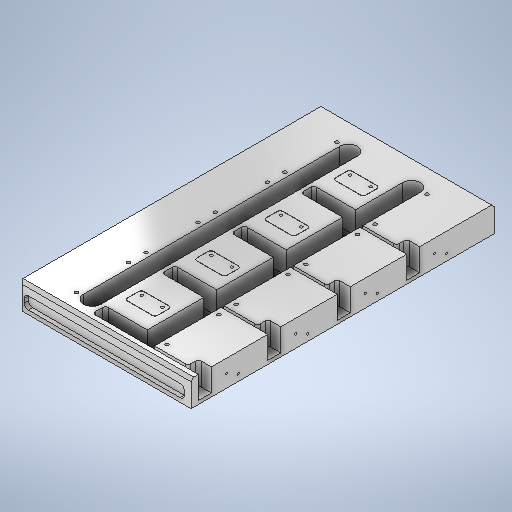
# Autodesk Inventor part: Assembly Plate
Saved by Autodesk Inventor 2025 (Build 290162000, 162)
## iProperties
Created: 2022-03-23
Part Number: Assembly Plate
Material: Generic
Document SubType Name: Modeling
Designer: Caleb
Density: 1 g/cm^3
Appearance: Aluminum - Dark
Author: Caleb
Autodesk Inventor part; units mm, degrees
ref_plane "YZ Plane" through (0, 0, 0) normal (1, 0, 0) x (0, 1, 0)
ref_plane "XZ Plane" through (0, 0, 0) normal (0, 1, 0) x (-1, 0, 0)
ref_plane "XY Plane" through (0, 0, 0) normal (0, 0, 1) x (1, 0, 0)
sketch "Sketch1" plane through (0, 0, 0) normal (0, 1, 0) x (-1, 0, 0)
  line L0 (-63.5, -111) -> (63.5, -111)
  line L1 (63.5, -111) -> (63.5, 111)
  line L2 (63.5, 111) -> (-63.5, 111)
  line L3 (-63.5, 111) -> (-63.5, -111)
  line L4 (-63.5, -111) -> (63.5, 111) construction
  line L5 (63.5, -111) -> (-63.5, 111) construction
  point P0 (0, 0)
  dimension "d0" = 127
  dimension "d1" = 222
  constraints: 12 end point, 2 midpoint, 2 parallel, 1 horizontal, 1 perpendicular
  measures "d0" distance of L2.end L1.end
  measures "d1" distance of L1.end L0.end
extrude "Extrusion1" add sketch "Sketch1" along normal blind 19.05
sketch "Sketch8" plane through (63.5, 0, -111) normal (0, 0, -1) x (-1, 0, 0)
  line L0 (119, 3) -> (8, 3)
  line L1 (5, 6) -> (5, 9)
  line L2 (8, 12) -> (119, 12)
  line L3 (122, 9) -> (122, 6)
  line L4 (122, 3) -> (5, 12) construction
  line L5 (5, 3) -> (122, 12) construction
  line L6 (0, 0) -> (0, 19.05) projected
  line L7 (127, 0) -> (127, 19.05) projected
  line L8 (0, 0) -> (127, 0) projected
  arc A0 (8, 12) -> (5, 9) centre (8, 9) ccw
  arc A1 (5, 6) -> (8, 3) centre (8, 6) ccw
  arc A2 (119, 3) -> (122, 6) centre (119, 6) ccw
  arc A3 (122, 9) -> (119, 12) centre (119, 9) ccw
  point P0 (63.5, 0)
  point P1 (63.5, 7.5)
  point P2 (0, 15.875)
  point P3 (127, 15.875)
  dimension "d77" = 9
  dimension "d78" = 5
  dimension "d79" = 5
  dimension "d80" = 3
  dimension "d83" = 3
  constraints: 12 end point, 8 point on circle, 8 point on line, 8 tangent, 4 centre point, 3 equal radius, 2 midpoint, 2 parallel, 1 horizontal, 1 perpendicular
  measures "d77" distance of L5.start L4.end
  measures "d78" distance between parallel lines of L6 L1
  measures "d79" distance between parallel lines of L7 L3
  measures "d80" distance between parallel lines of L8 L0
  measures "d83" radius of A0
extrude "Extrusion4" cut sketch "Sketch8" against normal blind 3
sketch "Sketch9" plane through (63.5, 0, 111) normal (0, 0, 1) x (1, 0, 0)
  line L0 (-8, 3) -> (-119, 3)
  line L1 (-122, 6) -> (-122, 9)
  line L2 (-119, 12) -> (-8, 12)
  line L3 (-5, 9) -> (-5, 6)
  line L4 (-5, 3) -> (-122, 12) construction
  line L5 (-122, 3) -> (-5, 12) construction
  arc A0 (-119, 12) -> (-122, 9) centre (-119, 9) ccw
  arc A1 (-122, 6) -> (-119, 3) centre (-119, 6) ccw
  arc A2 (-8, 3) -> (-5, 6) centre (-8, 6) ccw
  arc A3 (-5, 9) -> (-8, 12) centre (-8, 9) ccw
  line L6 (-127, 0) -> (0, 0) projected
  line L7 (-127, 0) -> (-127, 19.05) projected
  line L8 (0, 0) -> (0, 19.05) projected
  point P0 (63.5, 0)
  point P1 (-63.5, 7.5)
  dimension "d84" = 9
  dimension "d88" = 3
  dimension "d89" = 3
  dimension "d93" = 5
  dimension "d94" = 5
  constraints: 12 end point, 8 point on circle, 8 point on line, 8 tangent, 4 centre point, 3 equal radius, 2 midpoint, 2 parallel, 1 horizontal, 1 perpendicular
  measures "d84" distance of L5.start L4.end
  measures "d88" radius of A0
  measures "d89" distance between parallel lines of L6 L0
  measures "d93" distance between parallel lines of L7 L1
  measures "d94" distance between parallel lines of L8 L3
extrude "Extrusion5" cut sketch "Sketch9" against normal blind 3
sketch "Sketch10" plane through (0, 19.05, 0) normal (0, 1, 0) x (1, 0, 0)
  line L0 (63.5, -111) -> (63.5, 111) projected
  line L1 (-63.5, -111) -> (63.5, -111) projected
  line L2 (-63.5, 111) -> (-63.5, -111) projected
  line L3 (13.3831, -79.25) -> (-9.5437, -79.25) construction
  line L4 (0, -90.2687) -> (0, -62.9539) construction
  line L5 (13.3831, -28.45) -> (-9.5437, -28.45) construction
  line L6 (0, -39.4687) -> (0, -12.1539) construction
  line L7 (13.3831, 22.35) -> (-9.5437, 22.35) construction
  line L8 (0, 11.3313) -> (0, 38.6461) construction
  line L9 (13.3831, 73.15) -> (-9.5437, 73.15) construction
  line L10 (0, 62.1313) -> (0, 89.4461) construction
  point P0 (23, -96.75)
  point P1 (23, -85.0833)
  point P2 (-23, -96.75)
  point P3 (-23, -85.0833)
  point P4 (23, -73.4167)
  point P5 (-23, -73.4167)
  point P6 (23, -61.75)
  point P7 (-23, -61.75)
  point P8 (0, -79.25)
  point P9 (33, -98.25)
  point P10 (33, -60.25)
  point P11 (-33, -98.25)
  point P12 (-33, -60.25)
  point P13 (0, -28.45)
  point P14 (-33, -9.45)
  point P15 (-33, -47.45)
  point P16 (33, -9.45)
  point P17 (33, -47.45)
  point P18 (-23, -10.95)
  point P19 (23, -10.95)
  point P20 (-23, -22.6167)
  point P21 (23, -22.6167)
  point P22 (-23, -34.2833)
  point P23 (-23, -45.95)
  point P24 (23, -34.2833)
  point P25 (23, -45.95)
  point P26 (0, 22.35)
  point P27 (-33, 41.35)
  point P28 (-33, 3.35)
  point P29 (33, 41.35)
  point P30 (33, 3.35)
  point P31 (-23, 39.85)
  point P32 (23, 39.85)
  point P33 (-23, 28.1833)
  point P34 (23, 28.1833)
  point P35 (-23, 16.5167)
  point P36 (-23, 4.85)
  point P37 (23, 16.5167)
  point P38 (23, 4.85)
  point P39 (0, 73.15)
  point P40 (-33, 92.15)
  point P41 (-33, 54.15)
  point P42 (33, 92.15)
  point P43 (33, 54.15)
  point P44 (-23, 90.65)
  point P45 (23, 90.65)
  point P46 (-23, 78.9833)
  point P47 (23, 78.9833)
  point P48 (-23, 67.3167)
  point P49 (-23, 55.65)
  point P50 (23, 67.3167)
  point P51 (23, 55.65)
  dimension "d96" = 14.25
  dimension "d97" = 11.6667
  dimension "d127" = 11.6667
  dimension "d128" = 11.6667
  dimension "d129" = 46
  dimension "d130" = 35
  dimension "d131" = 17.5
  dimension "d132" = 23
  dimension "d133" = 33
  dimension "d134" = 19
  dimension "d135" = 38
  dimension "d136" = 33
  dimension "d146" = 50.8
  dimension "d154" = 63.5
  dimension "d155" = 127
  constraints: 16 end point, 8 point on line, 8 vertical alignment, 6 horizontal alignment, 2 perpendicular, 2 vertical, 1 horizontal, 57 other
  measures "d96" distance from line of point (23, -96.75) L1
  measures "d97" distance of point (23, -96.75) point (23, -85.083)
  measures "d127" distance of point (23, -85.083) point (23, -73.417)
  measures "d128" distance of point (23, -73.417) point (23, -61.75)
  measures "d129" distance of point (23, -96.75) point (-23, -96.75)
  measures "d130" distance of point (-23, -96.75) point (-23, -61.75)
  measures "d131" distance from line of point (-23, -61.75) L3
  measures "d132" distance from line of point (-23, -96.75) L4
  measures "d133" horizontal distance of point (33, -98.25) point (0, -79.25)
  measures "d134" vertical distance of point (33, -98.25) point (0, -79.25)
  measures "d135" distance of point (33, -60.25) point (33, -98.25)
  measures "d136" horizontal distance of point (-33, -98.25) point (0, -79.25)
  measures "d146" distance of L3.start L5.start
  measures "d154" distance from line of L0 point (0, -79.25)
  measures "d155" distance of L1.start L0.start
chamfer "Chamfer3" distance 2 angle 45 3 edges at (0, 19.05, 111) (-63.5, 19.05, 0) (0, 19.05, -111)
hole "Hole6" at (-33, 19.05, 98.25) at (-33, 19.05, 60.25) at (33, 19.05, 60.25) at (33, 19.05, 98.25) at (33, 19.05, -54.15) at (33, 19.05, -92.15) at (33, 19.05, -3.35) at (33, 19.05, -41.35) at (33, 19.05, 47.45) at (33, 19.05, 9.45) at (-33, 19.05, -54.15) at (-33, 19.05, -92.15) at (-33, 19.05, -3.35) at (-33, 19.05, -41.35) at (-33, 19.05, 47.45) at (-33, 19.05, 9.45) direction (0, -1, 0) diameter 2.459 end through all thread size "M3x0.5" class "6H" standard "ANSI Metric M Profile"
chamfer "Chamfer4" distance 4 angle 45 1 edges at (-63.5, 8.525, 111)
sketch "Sketch16" plane through (0, 19.05, 0) normal (0, 1, 0) x (1, 0, 0)
  circle A0 centre (-33, -60.25) radius 1.2295 projected
  circle A1 centre (-33, -98.25) radius 1.2295 projected
  line L0 (-61.5, -109) -> (-61.5, 109) projected
  circle A2 centre (-33, -47.45) radius 1.2295 projected
  point P0 (0, 0)
  point P1 (7.5, -75.95)
  point P2 (-7.5, -75.95)
  point P3 (-7.5, -25.15)
  point P4 (7.5, -25.15)
  point P5 (-7.5, 25.65)
  point P6 (7.5, 25.65)
  point P7 (-7.5, 76.45)
  point P8 (7.5, 76.45)
  dimension "d217" = 15
  dimension "d249" = 7.5
  dimension "d251" = 38
  dimension "d252" = 22.3
  dimension "d253" = 50.8
  dimension "d256" = 50.8
  constraints: 1 horizontal alignment, 1 vertical, 6 other
  measures "d217" distance of point (-7.5, -75.95) point (7.5, -75.95)
  measures "d249" horizontal distance of point (-7.5, -75.95) point (0, 0)
  measures "d251" distance of A0.centre A1.centre
  measures "d252" vertical distance of A1.centre point (-7.5, -75.95)
  measures "d253" distance of A2.centre A1.centre
  measures "d256" distance of point (-7.5, -75.95) point (-7.5, -25.15)
hole "Hole8" at (7.5, 19.05, 75.95) at (-7.5, 19.05, 75.95) at (7.5, 19.05, -76.45) at (-7.5, 19.05, -76.45) at (7.5, 19.05, -25.65) at (-7.5, 19.05, -25.65) at (7.5, 19.05, 25.15) at (-7.5, 19.05, 25.15) direction (0, -1, 0) diameter 2 end through all
sketch "Sketch19" plane through (0, 19.05, 0) normal (0, 1, 0) x (1, 0, 0)
  line L0 (-9, -84.95) -> (9, -84.95)
  line L1 (11, -82.95) -> (11, -74.95)
  line L2 (9, -72.95) -> (-9, -72.95)
  line L3 (-11, -74.95) -> (-11, -82.95)
  line L4 (-11, -84.95) -> (11, -72.95) construction
  line L5 (11, -84.95) -> (-11, -72.95) construction
  circle A0 centre (-7.5, -75.95) radius 1 projected
  arc A1 (-9, -72.95) -> (-11, -74.95) centre (-9, -74.95) ccw
  arc A2 (-11, -82.95) -> (-9, -84.95) centre (-9, -82.95) ccw
  arc A3 (9, -84.95) -> (11, -82.95) centre (9, -82.95) ccw
  arc A4 (11, -74.95) -> (9, -72.95) centre (9, -74.95) ccw
  circle A5 centre (-7.5, -25.15) radius 1 projected
  arc A6 (9, -34.15) -> (11, -32.15) centre (9, -32.15) ccw
  line L6 (11, -32.15) -> (11, -24.15)
  arc A7 (11, -24.15) -> (9, -22.15) centre (9, -24.15) ccw
  line L7 (-9, -34.15) -> (9, -34.15)
  arc A8 (-11, -32.15) -> (-9, -34.15) centre (-9, -32.15) ccw
  line L8 (-11, -34.15) -> (11, -22.15) construction
  line L9 (11, -34.15) -> (-11, -22.15) construction
  line L10 (9, -22.15) -> (-9, -22.15)
  arc A9 (-9, -22.15) -> (-11, -24.15) centre (-9, -24.15) ccw
  line L11 (-11, -24.15) -> (-11, -32.15)
  arc A10 (9, 16.65) -> (11, 18.65) centre (9, 18.65) ccw
  line L12 (11, 18.65) -> (11, 26.65)
  arc A11 (11, 26.65) -> (9, 28.65) centre (9, 26.65) ccw
  line L13 (-9, 16.65) -> (9, 16.65)
  arc A12 (-11, 18.65) -> (-9, 16.65) centre (-9, 18.65) ccw
  line L14 (-11, 16.65) -> (11, 28.65) construction
  line L15 (11, 16.65) -> (-11, 28.65) construction
  line L16 (9, 28.65) -> (-9, 28.65)
  arc A13 (-9, 28.65) -> (-11, 26.65) centre (-9, 26.65) ccw
  line L17 (-11, 26.65) -> (-11, 18.65)
  arc A14 (9, 67.45) -> (11, 69.45) centre (9, 69.45) ccw
  line L18 (11, 69.45) -> (11, 77.45)
  arc A15 (11, 77.45) -> (9, 79.45) centre (9, 77.45) ccw
  line L19 (-9, 67.45) -> (9, 67.45)
  arc A16 (-11, 69.45) -> (-9, 67.45) centre (-9, 69.45) ccw
  line L20 (-11, 67.45) -> (11, 79.45) construction
  line L21 (11, 67.45) -> (-11, 79.45) construction
  line L22 (9, 79.45) -> (-9, 79.45)
  arc A17 (-9, 79.45) -> (-11, 77.45) centre (-9, 77.45) ccw
  line L23 (-11, 77.45) -> (-11, 69.45)
  point P0 (0, 0)
  point P1 (0, -78.95)
  point P2 (0, -28.15)
  point P3 (0, 22.65)
  point P4 (0, 73.45)
  dimension "d281" = 3
  dimension "d282" = 9
  dimension "d283" = 22
  dimension "d284" = 2
  dimension "d285" = 50.8
  dimension "d288" = 50.8
  constraints: 48 end point, 32 point on circle, 32 point on line, 16 centre point, 8 tangent, 3 equal radius, 2 midpoint, 2 parallel, 1 collinear, 1 horizontal, 1 perpendicular, 1 vertical, 1 vertical alignment, 80 other
  measures "d281" distance from line of A0.centre L2
  measures "d282" distance from line of L0 A0.centre
  measures "d283" distance between parallel lines of L1 L3
  measures "d284" radius of A1
  measures "d285" distance of A5.centre A0.centre
  measures "d288" distance of L1.start L6.start
extrude "Extrusion13" cut sketch "Sketch19" against normal blind 0.2
hole "Hole5" at (23, 19.05, 96.75) at (23, 19.05, 85.0833) at (-23, 19.05, 96.75) at (-23, 19.05, 85.0833) at (23, 19.05, 73.4167) at (23, 19.05, 61.75) at (-23, 19.05, 61.75) at (-23, 19.05, 73.4167) at (-23, 19.05, -55.65) at (-23, 19.05, -67.3167) at (-23, 19.05, -78.9833) at (-23, 19.05, -90.65) at (-23, 19.05, -4.85) at (-23, 19.05, -16.5167) at (-23, 19.05, -28.1833) at (-23, 19.05, -39.85) at (-23, 19.05, 45.95) at (-23, 19.05, 34.2833) at (-23, 19.05, 22.6167) at (-23, 19.05, 10.95) at (23, 19.05, -55.65) at (23, 19.05, -67.3167) at (23, 19.05, -78.9833) at (23, 19.05, -90.65) at (23, 19.05, -4.85) at (23, 19.05, -16.5167) at (23, 19.05, -28.1833) at (23, 19.05, -39.85) at (23, 19.05, 45.95) at (23, 19.05, 34.2833) at (23, 19.05, 22.6167) at (23, 19.05, 10.95) direction (0, -1, 0) diameter 3.9624 end through all counterbore diameter 12.7 counterbore depth 15.5 thread size "10-32 UNF" class "2B" standard "ANSI Unified Screw Threads"
sketch "Sketch18" plane through (0, 19.05, 0) normal (0, 1, 0) x (1, 0, 0)
  line L0 (16.65, 90.65) -> (16.65, -104.15)
  line L1 (29.35, -104.15) -> (29.35, 90.65)
  arc A0 (20.4911, -90.9167) -> (25.5089, -90.9167) centre (23, -96.75) ccw projected
  arc A1 (25.5089, 84.8167) -> (20.4911, 84.8167) centre (23, 90.65) ccw projected
  line L2 (-29.35, 90.65) -> (-29.35, -96.75)
  line L3 (-16.65, -96.75) -> (-16.65, 90.65)
  arc A2 (-20.4911, -90.9167) -> (-20.4911, -79.25) centre (-23, -85.0833) ccw projected
  arc A3 (-25.5089, -79.25) -> (-25.5089, -90.9167) centre (-23, -85.0833) ccw projected
  arc A4 (-25.5089, -90.9167) -> (-20.4911, -90.9167) centre (-23, -96.75) ccw projected
  arc A5 (-20.4911, 84.8167) -> (-25.5089, 84.8167) centre (-23, 90.65) ccw projected
  line L4 (16.65, -104.15) -> (29.35, -104.15)
  point P0 (0, 0)
  point P1 (16.65, -96.75)
  point P2 (29.35, -96.75)
  constraints: 10 end point, 6 point on circle, 4 tangent, 2 parallel, 1 perpendicular
extrude "Extrusion12" cut sketch "Sketch18" against normal blind 16.5
sketch "Sketch17" plane through (0, 19.05, 0) normal (0, 1, 0) x (1, 0, 0)
  line L0 (-12, -105.65) -> (26, -105.65)
  line L1 (26, -101.65) -> (26, -98.15)
  line L2 (24, -96.15) -> (-12, -96.15)
  line L3 (-14, -98.15) -> (-14, -103.65)
  line L4 (63.5, -111) -> (63.5, 111) projected
  line L5 (63.5, -105.65) -> (54, -105.65)
  line L6 (54, -101.65) -> (54, -98.15)
  line L7 (56, -96.15) -> (63.5, -96.15)
  line L8 (63.5, -96.15) -> (63.5, -105.65)
  circle A0 centre (-33, -47.45) radius 1.2295 projected
  circle A1 centre (-33, -98.25) radius 1.2295 projected
  line L9 (26, -105.65) -> (54, -105.65)
  line L10 (28, -103.65) -> (52, -103.65)
  arc A2 (-12, -96.15) -> (-14, -98.15) centre (-12, -98.15) ccw
  arc A3 (26, -98.15) -> (24, -96.15) centre (24, -98.15) ccw
  arc A4 (-14, -103.65) -> (-12, -105.65) centre (-12, -103.65) ccw
  arc A5 (26, -101.65) -> (28, -103.65) centre (28, -101.65) ccw
  arc A6 (52, -103.65) -> (54, -101.65) centre (52, -101.65) ccw
  arc A7 (56, -96.15) -> (54, -98.15) centre (56, -98.15) ccw
  line L11 (54, -50.85) -> (54, -47.35)
  line L12 (56, -45.35) -> (63.5, -45.35)
  line L13 (63.5, -45.35) -> (63.5, -54.85)
  arc A8 (56, -45.35) -> (54, -47.35) centre (56, -47.35) ccw
  line L14 (28, -52.85) -> (52, -52.85)
  line L15 (26, -54.85) -> (54, -54.85)
  arc A9 (26, -50.85) -> (28, -52.85) centre (28, -50.85) ccw
  arc A10 (26, -47.35) -> (24, -45.35) centre (24, -47.35) ccw
  line L16 (26, -50.85) -> (26, -47.35)
  line L17 (63.5, -54.85) -> (54, -54.85)
  arc A11 (52, -52.85) -> (54, -50.85) centre (52, -50.85) ccw
  line L18 (-12, -54.85) -> (26, -54.85)
  line L19 (24, -45.35) -> (-12, -45.35)
  line L20 (-14, -47.35) -> (-14, -52.85)
  arc A12 (-14, -52.85) -> (-12, -54.85) centre (-12, -52.85) ccw
  arc A13 (-12, -45.35) -> (-14, -47.35) centre (-12, -47.35) ccw
  line L21 (54, -0.05) -> (54, 3.45)
  line L22 (56, 5.45) -> (63.5, 5.45)
  line L23 (63.5, 5.45) -> (63.5, -4.05)
  arc A14 (56, 5.45) -> (54, 3.45) centre (56, 3.45) ccw
  line L24 (28, -2.05) -> (52, -2.05)
  line L25 (26, -4.05) -> (54, -4.05)
  arc A15 (26, -0.05) -> (28, -2.05) centre (28, -0.05) ccw
  arc A16 (26, 3.45) -> (24, 5.45) centre (24, 3.45) ccw
  line L26 (26, -0.05) -> (26, 3.45)
  line L27 (63.5, -4.05) -> (54, -4.05)
  arc A17 (52, -2.05) -> (54, -0.05) centre (52, -0.05) ccw
  line L28 (-12, -4.05) -> (26, -4.05)
  line L29 (24, 5.45) -> (-12, 5.45)
  line L30 (-14, 3.45) -> (-14, -2.05)
  arc A18 (-14, -2.05) -> (-12, -4.05) centre (-12, -2.05) ccw
  arc A19 (-12, 5.45) -> (-14, 3.45) centre (-12, 3.45) ccw
  line L31 (54, 50.75) -> (54, 54.25)
  line L32 (56, 56.25) -> (63.5, 56.25)
  line L33 (63.5, 56.25) -> (63.5, 46.75)
  arc A20 (56, 56.25) -> (54, 54.25) centre (56, 54.25) ccw
  line L34 (28, 48.75) -> (52, 48.75)
  line L35 (26, 46.75) -> (54, 46.75)
  arc A21 (26, 50.75) -> (28, 48.75) centre (28, 50.75) ccw
  arc A22 (26, 54.25) -> (24, 56.25) centre (24, 54.25) ccw
  line L36 (26, 50.75) -> (26, 54.25)
  line L37 (63.5, 46.75) -> (54, 46.75)
  arc A23 (52, 48.75) -> (54, 50.75) centre (52, 50.75) ccw
  line L38 (-12, 46.75) -> (26, 46.75)
  line L39 (24, 56.25) -> (-12, 56.25)
  line L40 (-14, 54.25) -> (-14, 48.75)
  arc A24 (-14, 48.75) -> (-12, 46.75) centre (-12, 48.75) ccw
  arc A25 (-12, 56.25) -> (-14, 54.25) centre (-12, 54.25) ccw
  point P0 (0, 0)
  point P1 (-14, -105.65)
  point P2 (26, -96.15)
  point P3 (-14, -96.15)
  point P4 (54, -96.15)
  point P5 (63.5, -96.15)
  point P6 (26, -103.65)
  point P7 (54, -103.65)
  point P8 (54, -52.85)
  point P9 (54, -45.35)
  point P10 (26, -52.85)
  point P11 (26, -45.35)
  point P12 (-14, -54.85)
  point P13 (-14, -45.35)
  point P14 (54, -2.05)
  point P15 (54, 5.45)
  point P16 (26, -2.05)
  point P17 (26, 5.45)
  point P18 (-14, -4.05)
  point P19 (-14, 5.45)
  point P20 (54, 48.75)
  point P21 (54, 56.25)
  point P22 (26, 48.75)
  point P23 (26, 56.25)
  point P24 (-14, 46.75)
  point P25 (-14, 56.25)
  dimension "d234" = 9.5
  dimension "d235" = 9.5
  dimension "d236" = 9.5
  dimension "d237" = 26
  dimension "d238" = 14
  dimension "d239" = 50.8
  dimension "d262" = 2
  dimension "d263" = 7.4
  dimension "d271" = 2
  dimension "d274" = 50.8
  constraints: 80 end point, 61 point on line, 48 point on circle, 24 centre point, 12 tangent, 5 equal radius, 4 parallel, 3 perpendicular, 2 horizontal, 1 collinear, 1 vertical, 131 other
  measures "d234" distance of point (-14, -96.15) point (-14, -105.65)
  measures "d235" distance of L5.end point (54, -96.15)
  measures "d236" distance of point (54, -96.15) L7.end
  measures "d237" distance from line of L1 point (0, 0)
  measures "d238" distance from line of point (0, 0) L3
  measures "d239" distance of A0.centre A1.centre
  measures "d262" distance between parallel lines of L9 L10
  measures "d263" distance from line of L0 A1.centre
  measures "d271" radius of A2
  measures "d274" distance of L6.start L11.start
extrude "Extrusion11" cut sketch "Sketch17" against normal blind 16.5 contours A4 L3 A2 L2 A3 L1 A5 L10 A6 L6 A7 L7 L4 L5 L9 L0 | L17 L15 L18 A12 L20 A13 L19 A10 L16 A9 L14 A11 L11 A8 L12 L4 | L27 L25 L28 A18 L30 A19 L29 A16 L26 A15 L24 A17 L21 A14 L22 L4 | L37 L35 L38 A24 L40 A25 L39 A22 L36 A21 L34 A23 L31 A20 L32 L4
sketch "Sketch20" plane through (63.5, 0, 111) normal (1, 0, 0) x (0, 0, -1)
  line L0 (14.85, 19.05) -> (14.85, 2.55) projected
  line L1 (0, 0) -> (222, 0) projected
  line L2 (65.65, 19.05) -> (65.65, 2.55) projected
  point P0 (111, 0)
  point P1 (34.535, 4.877)
  point P2 (25.823, 9.246)
  point P3 (14.85, 3.55)
  point P4 (65.65, 3.55)
  point P5 (85.335, 4.877)
  point P6 (76.623, 9.246)
  point P7 (136.135, 4.877)
  point P8 (127.423, 9.246)
  point P9 (186.935, 4.877)
  point P10 (178.223, 9.246)
  dimension "d295" = 10.973
  dimension "d296" = 19.685
  dimension "d297" = 9.246
  dimension "d298" = 4.877
  dimension "d299" = 50.8
  dimension "d302" = 50.8
  constraints: 1 horizontal, 6 other
  measures "d295" distance from line of point (25.823, 9.246) L0
  measures "d296" distance from line of L0 point (34.535, 4.877)
  measures "d297" distance from line of L1 point (25.823, 9.246)
  measures "d298" distance from line of point (34.535, 4.877) L1
  measures "d299" distance between parallel lines of L0 L2
  measures "d302" distance of point (34.535, 4.877) point (85.335, 4.877)
hole "Hole9" at (63.5, 4.877, 76.465) at (63.5, 9.246, 85.177) at (63.5, 4.877, 25.665) at (63.5, 9.246, 34.377) at (63.5, 4.877, -25.135) at (63.5, 9.246, -16.423) at (63.5, 4.877, -75.935) at (63.5, 9.246, -67.223) direction (-1, 0, 0) diameter 1.567 depth 6.3 tip angle 118 thread size "M2x0.4" class "6H" standard "ANSI Metric M Profile"
equation "\"d79\" = d78"
equation "\"d128\" = d97"
equation "\"d131\" = 0.5 * d130"
equation "\"d132\" = 0.5 * d129"
equation "\"d135\" = 2 * d134"
equation "\"d136\" = d133"
equation "\"d154\" = 0.5 * d155"
body "Solid1"
